slot_gauge (Autodesk Fusion 360 design; units mm, degrees)
part number: 2026-09-02-15-56-11-666
Autodesk Fusion 360 part; units mm, degrees
sketch "Plate" plane through (0, 0, 0) normal (0, 1, 0) x (1, 0, 0)
  line L0 (0, 0) -> (5, 0)
  line L1 (5, 0) -> (5, -90)
  line L2 (5, -90) -> (0, -90)
  line L3 (0, -90) -> (0, 0)
  dimension "d67" = 5
  dimension "d68" = 90
  constraint coincident L0.start L3.end
  constraint horizontal L0
  constraint horizontal L2
  constraint vertical L1
  constraint vertical L3
  measures "d67" horizontal distance of L0.start L1.end
  measures "d68" vertical distance of L0.start L1.end
extrude "Plate (1)" add sketch "Plate" along normal mid plane 24
sketch "Hook profile" plane through (0, 0, 0) normal (0, 1, 0) x (1, 0, 0)
  line L0 (0, -88) -> (-8.3, -88)
  line L1 (-8.3, -88) -> (-8.3, -71)
  line L2 (-8.3, -71) -> (-5.3, -71)
  line L3 (-5.3, -71) -> (-3.8, -72.5)
  line L4 (-3.8, -72.5) -> (-3.8, -83)
  line L5 (-3.8, -83) -> (0, -83)
  line L6 (0, -83) -> (0, -88)
  dimension "d71" = 88
  dimension "d72" = 8.3
  dimension "d73" = 3.8
  dimension "d74" = 5
  dimension "d75" = 10.5
  dimension "d76" = 1.5
  dimension "d77" = 1.5
  constraint horizontal L0
  constraint horizontal L2
  constraint horizontal L5
  constraint vertical L1
  constraint vertical L4
  constraint vertical L6
  constraint coincident origin L6
  measures "d71" vertical distance of origin L0.start
  measures "d72" horizontal distance of L0.start L0.end
  measures "d73" horizontal distance of L4.end L5.end
  measures "d74" vertical distance of L0.start L5.end
  measures "d75" vertical distance of L3.end L4.end
  measures "d76" horizontal distance of L2.end L3.end
  measures "d77" vertical distance of L2.end L3.end
extrude "Hook profile (1)" add sketch "Hook profile" along normal mid plane 2.4
pattern_linear "Hook rows" count 4 spacing 25.4 along (0, 0, -1) count 3 spacing 0 along (0, 0, 1) of "Hook profile (1)"
equation "bracketWidth = 24.0 mm" comment "gauge width, as the bracket"
equation "hookTabWidth = slotWidth - 0.8 mm" comment "blade width through the slot"
equation "slotPitchVertical = 25.4 mm" comment "1 inch, measured"
equation "slotWidth = 3.2 mm" comment "measured slot width in the upright"
equation "faceMetalThickness = 2.0 mm" comment "upright face metal"
equation "hookThroat = faceMetalThickness + 1.8 mm" comment "gap behind the plate"
equation "hookNeckHeight = 5.0 mm" comment "bears on the slot bottom edge"
equation "hookLipThickness = 4.5 mm" comment "lip thickness behind the face"
equation "hookLipDrop = 12.0 mm" comment "engagement below the neck"
equation "plateHeight = 90.0 mm" comment "plate height"
equation "gaugePlateThickness = 5.0 mm" comment "gauge plate"
equation "hookLipChamfer = 1.5 mm" comment "lead-in past slot burrs"
equation "topHookNeckTop = 88.0 mm" comment "top row, below the plate top"
equation "hookRows = 4" comment "number of hook rows (pattern count)"
equation "d67 = gaugePlateThickness"
equation "d68 = plateHeight"
equation "d69 = bracketWidth"
equation "d71 = topHookNeckTop"
equation "d72 = hookThroat + hookLipThickness"
equation "d73 = hookThroat"
equation "d74 = hookNeckHeight"
equation "d75 = hookLipDrop - hookLipChamfer"
equation "d76 = hookLipChamfer"
equation "d77 = hookLipChamfer"
equation "d78 = hookTabWidth"
equation "d80 = hookRows"
equation "d82 = -slotPitchVertical"
named bodies: "slot_gauge"
